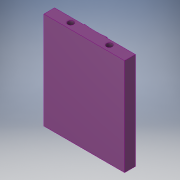
# Autodesk Inventor part: joint3_rot_con
Saved by Autodesk Inventor 2019 (Build 230136000, 136)
## iProperties
Created: 2019-12-29
Part Number: joint3_rot_con
Material: Пластик АБС
Document SubType Name: Modeling
Designer: Петров Иван
Density: 1.06 g/cm^3
Appearance: Гладкий — пурпурный
Author: Петров Иван
Autodesk Inventor part; units mm, degrees
ref_plane "YZ Plane" through (0, 0, 0) normal (1, 0, 0) x (0, 1, 0)
ref_plane "XZ Plane" through (0, 0, 0) normal (0, 1, 0) x (-1, 0, 0)
ref_plane "XY Plane" through (0, 0, 0) normal (0, 0, 1) x (1, 0, 0)
sketch "Эскиз1" plane through (0, 0, 0) normal (0, 1, 0) x (-1, 0, 0)
  arc A0 (4.0194, -3.1709) -> (-7.7806, -3.1709) centre (-1.8806, -45.2594) ccw
  line L0 (-7.7806, -3.1709) -> (-7.7806, 2.8291)
  line L1 (-7.7806, 2.8291) -> (4.0194, 2.8291)
  line L2 (4.0194, 2.8291) -> (4.0194, -3.1709)
  point P0 (0, -39)
  dimension "d1" = 6
  dimension "d12" = 11.8
  constraints: 6 end point, 2 perpendicular, 2 point on circle, 1 centre point, 1 vertical
  measures "d1" distance of L0.start L0.end
  measures "d12" distance of L0.end L1.end
extrude "Выдавливание1" add sketch "Эскиз1" along normal blind 50.2
sketch "Эскиз4" plane through (0, 0, 0) normal (0, -1, 0) x (1, 0, 0)
  arc A0 (7.7806, -3.1709) -> (-4.0194, -3.1709) centre (1.8806, -45.2594) ccw projected
  line L0 (1.8806, -2.7594) -> (-4.0194, -2.7594)
  line L1 (-4.0194, -3.1709) -> (-4.0194, 2.8291) projected
  line L2 (-4.0194, 2.8291) -> (-19.0194, 2.8291)
  line L3 (-19.0194, 2.8291) -> (-19.0194, -2.7594)
  line L4 (-19.0194, -2.7594) -> (-4.0194, -2.7594)
  line L5 (-4.0194, -2.7594) -> (-4.0194, 2.8291)
  line L6 (7.7806, 2.8291) -> (7.7806, -3.1709) projected
  line L7 (7.7806, 2.8291) -> (22.7806, 2.8291)
  line L8 (22.7806, 2.8291) -> (22.7806, -2.7594)
  line L9 (22.7806, -2.7594) -> (7.7806, -2.7594)
  line L10 (7.7806, -2.7594) -> (7.7806, 2.8291)
  point P0 (0, 0)
  dimension "d13" = 15
  dimension "d16" = 15
  constraints: 18 end point, 4 parallel, 3 horizontal, 2 perpendicular, 1 point on circle, 1 point on line
  measures "d13" distance of L4.end L3.end
  measures "d16" distance of L8.end L9.end
extrude "Выдавливание4" add sketch "Эскиз4" against normal up to surface (50.2 mm away) contours L4 L3 L2 L1 | L7 L8 L9 L6
sketch "Эскиз5" plane through (0, 0, 0) normal (0, -1, 0) x (1, 0, 0)
  line L0 (22.7806, 2.8291) -> (-19.0194, 2.8291) projected
  line L1 (1.8806, 2.8291) -> (1.8806, -0.1709)
  line L2 (1.8806, -0.1709) -> (-8.1194, -0.1709)
  line L3 (-8.1194, -0.1709) -> (11.8806, -0.1709)
  circle A0 centre (-8.1194, -0.1709) radius 1.5
  circle A1 centre (11.8806, -0.1709) radius 1.5
  point P0 (0, 0)
  dimension "d17" = 3
  dimension "d18" = 10
  dimension "d19" = 20
  dimension "d20" = 3
  dimension "d21" = 3
  constraints: 6 end point, 2 centre point, 2 coincident, 1 midpoint, 1 perpendicular, 1 point on line, 1 vertical
  measures "d17" distance of L1.start L1.end
  measures "d18" distance of L1.end L2.end
  measures "d19" distance of L2.end L3.end
  measures "d20" diameter of A0
  measures "d21" diameter of A1
extrude "Выдавливание5" cut sketch "Эскиз5" against normal blind 10
sketch "Эскиз6" plane through (0, 50.2, 0) normal (0, 1, 0) x (1, 0, 0)
  circle A0 centre (-8.1194, 0.1709) radius 1.5 projected
  circle A1 centre (-8.1194, 0.1709) radius 1.5
  circle A2 centre (11.8806, 0.1709) radius 1.5 projected
  circle A3 centre (11.8806, 0.1709) radius 1.5
  point P0 (0, 0)
  constraints: 2 centre point, 2 coincident
extrude "Выдавливание6" cut sketch "Эскиз6" against normal blind 10
